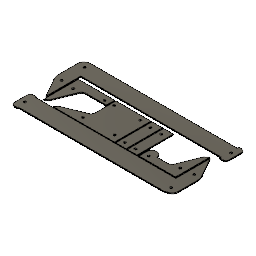
caliperModelOnly (Autodesk Fusion 360 design; units mm, degrees)
Autodesk Fusion 360 part; units mm, degrees
sketch "Sketch1" plane through (0, 0, 0) normal (0, 0, 1) x (1, 0, 0) in component "Component"
  line L0 (21.310022, 39.904503) -> (21.310022, 94.903812)
  line L1 (3.945382, 70.29264) -> (21.310022, 39.904503)
  arc A0 (3.945382, 70.29264) -> (1.310278, 80.215262) centre (21.310026, 80.215294) cw
  line L2 (1.310279, 109.903612) -> (1.310278, 80.215262)
  arc A1 (1.310279, 109.903612) -> (11.310152, 119.903488) centre (11.310152, 109.903615) cw
  line L3 (241.184429, 119.907462) -> (11.310152, 119.903488)
  line L4 (241.184429, 122.407407) -> (241.184429, 119.907462)
  line L5 (246.184367, 122.407407) -> (241.184429, 122.407407)
  arc A2 (246.184367, 122.407407) -> (251.184306, 117.407452) centre (246.184369, 117.40747) cw
  line L6 (251.184306, 97.40773) -> (251.184306, 117.407452)
  arc A3 (251.184306, 97.40773) -> (246.184367, 92.407775) centre (246.184369, 97.407711) cw
  line L7 (241.184429, 92.407775) -> (246.184367, 92.407775)
  line L8 (241.184429, 94.907752) -> (241.184429, 92.407775)
  line L9 (42.661135, 72.402174) -> (29.049648, 38.492042)
  line L10 (80.737159, 89.049624) -> (80.737159, 75.459087)
  line L11 (23.416198, 89.049624) -> (80.737159, 89.049624)
  line L12 (23.416198, 34.050315) -> (23.416198, 89.049624)
  line L13 (21.310022, 94.903812) -> (241.184429, 94.907752)
  line L14 (80.737159, 75.459087) -> (48.944918, 75.459055)
  arc A4 (42.661118, 72.402151) -> (48.945273, 75.459055) centre (48.623841, 68.132131) cw
  line L15 (23.416198, 34.050315) -> (29.049648, 38.492042)
  arc A5 (30.390951, 72.141115) -> (33.790907, 72.141115) centre (32.090929, 72.142719) cw
  arc A6 (33.790907, 72.141115) -> (30.390951, 72.141115) centre (32.090929, 72.13951) cw
  arc A7 (74.649025, 80.478227) -> (71.249066, 80.478227) centre (72.949045, 80.478227) cw
  arc A8 (71.249066, 80.478227) -> (74.649025, 80.478227) centre (72.949045, 80.478227) cw
  line L16 (155.459087, 31.728651) -> (155.459087, 89.049624)
  line L17 (138.934303, 31.728651) -> (155.459087, 31.728651)
  arc A9 (144.095518, 79.228028) -> (147.495478, 79.228028) centre (145.795498, 79.228028) cw
  arc A10 (147.495478, 79.228028) -> (144.095518, 79.228028) centre (145.795498, 79.228028) cw
  arc A11 (144.095518, 39.228551) -> (147.495478, 39.228551) centre (145.795498, 39.228551) cw
  arc A12 (147.495478, 39.228551) -> (144.095518, 39.228551) centre (145.795498, 39.228551) cw
  line L18 (138.934303, 89.049624) -> (138.934303, 31.728651)
  line L19 (155.459087, 89.049624) -> (138.934303, 89.049624)
  line L20 (137.369851, 89.049624) -> (137.369851, 31.728651)
  line L21 (120.845066, 89.049624) -> (137.369851, 89.049624)
  arc A13 (126.006274, 41.550247) -> (129.406233, 41.550247) centre (127.706254, 41.550247) cw
  arc A14 (129.406233, 41.550247) -> (126.006274, 41.550247) centre (127.706254, 41.550247) cw
  arc A15 (126.006274, 81.549724) -> (129.406233, 81.549724) centre (127.706254, 81.549724) cw
  arc A16 (129.406233, 81.549724) -> (126.006274, 81.549724) centre (127.706254, 81.549724) cw
  line L22 (137.369851, 31.728651) -> (120.845066, 31.728651)
  arc A17 (85.57402, 81.261503) -> (88.97398, 81.261503) centre (87.274, 81.261503) cw
  arc A18 (88.97398, 81.261503) -> (85.57402, 81.261503) centre (87.274, 81.261503) cw
  arc A19 (80.636859, 40.403368) -> (77.2369, 40.403368) centre (78.93688, 40.403368) cw
  arc A20 (77.2369, 40.403368) -> (80.636859, 40.403368) centre (78.93688, 40.403368) cw
  arc A21 (82.254852, 57.257392) -> (79.197931, 50.973584) centre (74.927929, 56.936301) cw
  line L23 (79.197931, 50.973584) -> (45.287815, 37.362087)
  line L24 (40.846072, 31.728651) -> (45.287815, 37.362087)
  line L25 (82.254852, 89.049624) -> (82.254852, 57.257392)
  line L26 (40.846072, 31.728651) -> (95.845381, 31.728651)
  line L27 (95.845381, 89.049624) -> (82.254852, 89.049624)
  line L28 (95.845381, 31.728651) -> (120.845066, 31.728651)
  line L29 (95.845381, 89.049624) -> (120.845066, 89.049624)
  line L30 (172.605838, 31.728651) -> (172.605838, 89.049624)
  line L31 (157.078186, 31.728651) -> (172.605838, 31.728651)
  arc A22 (161.242253, 79.228028) -> (164.642213, 79.228028) centre (162.942233, 79.228028) cw
  arc A23 (164.642213, 79.228028) -> (161.242253, 79.228028) centre (162.942233, 79.228028) cw
  arc A24 (161.242253, 39.228551) -> (164.642213, 39.228551) centre (162.942233, 39.228551) cw
  arc A25 (164.642213, 39.228551) -> (161.242253, 39.228551) centre (162.942233, 39.228551) cw
  line L32 (157.078186, 89.049624) -> (157.078186, 31.728651)
  line L33 (172.605838, 89.049624) -> (157.078186, 89.049624)
  arc A26 (184.669194, 39.743533) -> (181.269235, 39.743533) centre (182.969214, 39.743533) cw
  arc A27 (181.269235, 39.743533) -> (184.669194, 39.743533) centre (182.969214, 39.743533) cw
  arc A28 (225.527297, 48.080613) -> (222.127337, 48.080613) centre (223.827317, 48.080613) cw
  arc A29 (222.127337, 48.080613) -> (225.527297, 48.080613) centre (223.827317, 48.080613) cw
  arc A30 (213.257125, 47.819585) -> (206.973333, 44.76264) centre (207.294392, 52.089565) cw
  line L34 (213.257125, 47.819585) -> (226.868606, 81.729685)
  line L35 (232.502058, 86.171412) -> (226.868606, 81.729685)
  line L36 (190.757328, 44.76264) -> (206.973333, 44.76264)
  line L37 (232.502058, 86.171412) -> (232.502058, 32.16922)
  line L38 (232.502058, 32.16922) -> (175.181101, 32.16922)
  line L39 (175.181101, 32.16922) -> (175.181101, 44.762608)
  line L40 (234.359511, 30.791285) -> (14.485117, 30.787312)
  line L41 (14.485117, 30.787312) -> (14.485111, 32.291271)
  line L42 (14.485111, 32.291271) -> (9.485179, 32.291271)
  arc A31 (4.48524, 27.291317) -> (9.485179, 32.291271) centre (9.485177, 27.291335) cw
  line L43 (4.48524, 27.291317) -> (4.485239, 7.291594)
  arc A32 (9.485177, 2.291672) -> (4.48524, 7.291594) centre (9.485177, 7.291608) cw
  line L44 (9.485177, 2.291672) -> (14.485111, 2.291672)
  line L45 (14.485111, 2.291672) -> (14.485111, 3.795534)
  line L46 (14.485111, 3.795534) -> (244.359389, 3.799506)
  arc A33 (254.359266, 14.795434) -> (244.359389, 4.795557) centre (244.359392, 14.795431) cw
  line L47 (254.359266, 14.795434) -> (254.359266, 44.483752)
  arc A34 (251.724156, 54.406439) -> (254.359266, 44.483752) centre (234.359517, 44.483775) cw
  line L48 (251.724156, 54.406439) -> (234.359511, 84.794576)
  line L49 (234.359511, 84.794576) -> (234.359511, 30.791285)
  arc A35 (13.665668, 74.301356) -> (10.265711, 74.301356) centre (11.96569, 74.301356) cw
  arc A36 (10.265711, 74.301356) -> (13.665668, 74.301356) centre (11.96569, 74.301356) cw
  arc A37 (13.985467, 110.118841) -> (10.58551, 110.118841) centre (12.285488, 110.118841) cw
  arc A38 (10.58551, 110.118841) -> (13.985467, 110.118841) centre (12.285488, 110.118841) cw
  arc A39 (244.880264, 108.519831) -> (241.480305, 108.519831) centre (243.180284, 108.519831) cw
  arc A40 (241.480305, 108.519831) -> (244.880264, 108.519831) centre (243.180284, 108.519831) cw
  arc A41 (245.403821, 50.39769) -> (242.003861, 50.39769) centre (243.703841, 50.39769) cw
  arc A42 (242.003861, 50.39769) -> (245.403821, 50.39769) centre (243.703841, 50.39769) cw
  arc A43 (245.084028, 14.580205) -> (241.684069, 14.580205) centre (243.384049, 14.580205) cw
  arc A44 (241.684069, 14.580205) -> (245.084028, 14.580205) centre (243.384049, 14.580205) cw
  arc A45 (14.189226, 16.179215) -> (10.789268, 16.179215) centre (12.489247, 16.179215) cw
  arc A46 (10.789268, 16.179215) -> (14.189226, 16.179215) centre (12.489247, 16.179215) cw
  arc A47 (190.757328, 44.76264) -> (175.181101, 44.76264) centre (182.969214, 44.76264) cw
  line L50 (244.359389, 4.795557) -> (244.359389, 3.799506)
  arc A48 (190.757328, 44.76264) -> (175.181101, 44.76264) centre (182.969214, 44.76264) ccw
extrude "Extrude1" add sketch "Sketch1" along normal blind 1.6 makes body 1 at (169.895179, 66.422903, 0) makes body 2 at (91.268201, 111.571587, 0) makes body 3 at (152.748434, 66.422903, 0) makes body 4 at (207.834842, 38.448765, 0) makes body 5 at (48.083414, 82.105335, 0) makes body 6 at (111.725004, 60.119121, 0) makes body 7 at (164.401337, 12.795442, 0) in component "Component"
component "Component" placed x (1, 0, 0) y (0, 1, 0) z (0, 0, 1) at (0, 0, 0)
